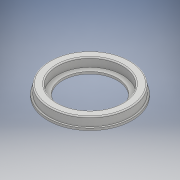
# Autodesk Inventor part: Mitutoyo-BD-black-ring
Saved by Autodesk Inventor 2017 (Build 210142000, 142)
## iProperties
Created: 2022-08-03
Part Number: Mitutoyo-BD-black-ring
Material: Generic
Document SubType Name: Modeling
Designer: Nikita
Density: 1 g/cm^3
Appearance: Default
Author: Nikita
Autodesk Inventor part; units mm, degrees
ref_plane "YZ Plane" through (0, 0, 0) normal (1, 0, 0) x (0, 1, 0)
ref_plane "XZ Plane" through (0, 0, 0) normal (0, 1, 0) x (-1, 0, 0)
ref_plane "XY Plane" through (0, 0, 0) normal (0, 0, 1) x (1, 0, 0)
sketch "Sketch1" plane through (0, 0, 0) normal (0, 0, 1) x (1, 0, 0)
  circle A0 centre (0, 0) radius 14.85
  circle A1 centre (0, 0) radius 18.5
  circle A2 centre (0, 0) radius 19.25
  circle A3 centre (0, 0) radius 12.5
  dimension "d0" = 29.7
  dimension "d1" = 37
  dimension "d2" = 38.5
  dimension "d8" = 25
  constraints: 4 centre point, 4 coincident
  measures "d0" diameter of A0
  measures "d1" diameter of A1
  measures "d2" diameter of A2
  measures "d8" diameter of A3
extrude "Extrusion1" add sketch "Sketch1" along normal blind 5 contours A1
extrude "Extrusion2" add sketch "Sketch1" along normal blind 1
fillet "Fillet1" radius 0.5 2 edges at (-14.85, 0, 5) (-18.5, 0, 5)
body "Solid1"
